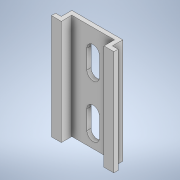
# Autodesk Inventor part: Part_B8
Saved by Autodesk Inventor 2022.6 (Build 266554010, 554A)
## iProperties
Created: 2025-06-02
Part Number: Part_B8
Material: Generic
Document SubType Name: Modeling
Designer: khinm
Density: 1 g/cm^3
Appearance: Default
Author: khinm
Autodesk Inventor part; units mm, degrees
ref_plane "YZ Plane" through (0, 0, 0) normal (1, 0, 0) x (0, 1, 0)
ref_plane "XZ Plane" through (0, 0, 0) normal (0, 1, 0) x (-1, 0, 0)
ref_plane "XY Plane" through (0, 0, 0) normal (0, 0, 1) x (1, 0, 0)
sketch "Sketch1" plane through (0, 0, 0) normal (0, 1, 0) x (-1, 0, 0)
  line L0 (14.85, 7) -> (10.15, 7)
  line L1 (10.15, 7) -> (10.15, 2)
  line L2 (10.15, 2) -> (-10.15, 2)
  line L3 (-10.15, 2) -> (-10.15, 7)
  line L4 (-10.15, 7) -> (-14.85, 7)
  line L5 (-14.85, 7) -> (-14.85, 5)
  line L6 (-14.85, 5) -> (-12.15, 5)
  line L7 (-12.15, 5) -> (-12.15, 0)
  line L8 (-12.15, 0) -> (12.15, 0)
  line L9 (12.15, 0) -> (12.15, 5)
  line L10 (12.15, 5) -> (14.85, 5)
  line L11 (14.85, 5) -> (14.85, 7)
  point P0 (0, 0)
  point P1 (0, 0)
  point P2 (0, 2)
  point P3 (12.5, 7)
  point P4 (13.5, 5)
  dimension "d0" = 20.3
  dimension "d1" = 24.3
  dimension "d2" = 5
  dimension "d3" = 4.7
  dimension "d5" = 2
  dimension "d6" = 2
  constraints: 24 end point, 8 perpendicular, 4 midpoint, 4 point on line, 2 collinear, 2 vertical alignment, 1 coincident, 1 horizontal, 1 parallel
  measures "d0" distance of L1.end L2.end
  measures "d1" distance of L7.end L8.end
  measures "d2" distance of L8.end L9.end
  measures "d3" distance of L0.start L0.end
  measures "d5" distance between parallel lines of L2 L8
  measures "d6" distance from line of L0 point (13.5, 5)
extrude "Extrusion1" add sketch "Sketch1" along normal mid plane 50
sketch "Sketch2" plane through (-10.15, 25, 2) normal (0, 0, 1) x (1, 0, 0)
  line L0 (13.1499, -10.0316) -> (13.1499, -19.0316)
  line L1 (7.1499, -19) -> (7.1499, -10)
  arc A0 (13.1499, -10.0316) -> (7.1499, -10) centre (10.15, -10) ccw
  arc A1 (7.1499, -19) -> (13.1499, -19.0316) centre (10.15, -19) ccw
  line L2 (0, 0) -> (20.3, 0) projected
  point P0 (10.15, -25)
  dimension "d9" = 6
  dimension "d12" = 9
  dimension "d13" = 10
  constraints: 4 end point, 4 point on circle, 2 centre point, 2 horizontal alignment, 2 parallel, 2 vertical alignment
  measures "d9" distance between parallel lines of L0 L1
  measures "d12" distance of L0.start L0.end
  measures "d13" distance from line of A0.centre L2
extrude "Extrusion2" cut sketch "Sketch2" against normal up to surface (2 mm away)
pattern_linear "Rectangular Pattern1" count 2 spacing 25 along (0, -1, 0) of "Extrusion2"
body "Solid1"
